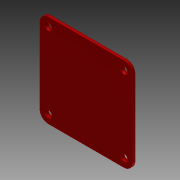
# Autodesk Inventor part: Durometer_Electronics_Enclosure
Saved by Autodesk Inventor 2015 (Build 190159000, 159)
## iProperties
Created: 2015-01-04
Part Number: Durometer_Electronics_Enclosure
Material: Generic
Document SubType Name: Modeling
Designer: Drew
Density: 1 g/cm^3
Appearance: Smooth - Red
Author: Drew
Autodesk Inventor part; units mm, degrees
ref_plane "YZ Plane" through (0, 0, 0) normal (1, 0, 0) x (0, 1, 0)
ref_plane "XZ Plane" through (0, 0, 0) normal (0, 1, 0) x (-1, 0, 0)
ref_plane "XY Plane" through (0, 0, 0) normal (0, 0, 1) x (1, 0, 0)
sketch "Sketch1" plane through (0, 0, 0) normal (0, 0, 1) x (1, 0, 0)
  line L0 (28.575, -34.925) -> (-28.575, -34.925)
  line L1 (-34.925, -28.575) -> (-34.925, 28.575)
  line L2 (-28.575, 34.925) -> (28.575, 34.925)
  line L3 (34.925, 28.575) -> (34.925, -28.575)
  line L4 (34.925, -34.925) -> (-34.925, 34.925) construction
  line L5 (-34.925, -34.925) -> (34.925, 34.925) construction
  arc A0 (-28.575, 34.925) -> (-34.925, 28.575) centre (-28.575, 28.575) ccw
  arc A1 (34.925, 28.575) -> (28.575, 34.925) centre (28.575, 28.575) ccw
  arc A2 (28.575, -34.925) -> (34.925, -28.575) centre (28.575, -28.575) ccw
  arc A3 (-34.925, -28.575) -> (-28.575, -34.925) centre (-28.575, -28.575) ccw
  point P0 (0, 0)
  dimension "d0" = 69.85
  dimension "d1" = 69.85
  dimension "d2" = 6.35
  constraints: 12 end point, 8 point on circle, 8 point on line, 8 tangent, 4 centre point, 3 equal radius, 2 midpoint, 2 parallel, 1 horizontal, 1 perpendicular
  measures "d0" distance of L4.end L5.end
  measures "d1" distance between parallel lines of L0 L2
  measures "d2" radius of A0
extrude "Extrusion1" add sketch "Sketch1" along normal blind 2.032
sketch "Sketch2" plane through (0, 0, 2.032) normal (0, 0, 1) x (1, 0, 0)
  arc A0 (-28.575, 34.925) -> (-34.925, 28.575) centre (-28.575, 28.575) ccw projected
  arc A1 (34.925, 28.575) -> (28.575, 34.925) centre (28.575, 28.575) ccw projected
  arc A2 (28.575, -34.925) -> (34.925, -28.575) centre (28.575, -28.575) ccw projected
  arc A3 (-34.925, -28.575) -> (-28.575, -34.925) centre (-28.575, -28.575) ccw projected
  point P0 (0, 0)
  constraints: 4 coincident
hole "Hole1" at (-28.575, 28.575, 2.032) at (28.575, 28.575, 2.032) at (28.575, -28.575, 2.032) at (-28.575, -28.575, 2.032) direction (0, 0, -1) diameter 3.2 end through all countersink diameter 5.6 countersink angle 90
sketch "Sketch3" plane through (0, 0, 0) normal (0, 0, -1) x (-1, 0, 0)
  circle A0 centre (14.605, 12.7) radius 1.3747
  circle A1 centre (-14.605, 12.7) radius 1.5
  point P0 (0, 0)
  dimension "d12" = 3
  dimension "d13" = 29.21
  dimension "d14" = 12.7
  dimension "d15" = 14.605
  constraints: 2 centre point
  measures "d12" diameter of A1
  measures "d13" distance of A0.centre A1.centre
  measures "d14" vertical distance of A0.centre point (0, 0)
  measures "d15" horizontal distance of point (0, 0) A0.centre
extrude "Extrusion2" add sketch "Sketch3" along normal blind 3.81
chamfer "Chamfer1" distance 0.508 angle 45 2 edges at (16.105, 12.7, -3.81) (-13.2303, 12.7, -3.81)
fillet "Fillet1" radius 1.27 2 edges at (-13.2303, 12.7, 0) (16.105, 12.7, 0)
equation "\"d0\" = d1"
body "Solid1"
